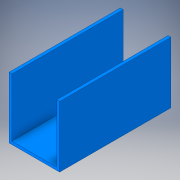
# Autodesk Inventor part: Hombro_base
Saved by Autodesk Inventor 2019 (Build 230136000, 136)
## iProperties
Created: 2020-02-08
Part Number: Hombro_base
Material: Generic
Document SubType Name: Modeling
Designer: Omar
Density: 1 g/cm^3
Appearance: Default
Author: Omar
Autodesk Inventor part; units mm, degrees
ref_plane "YZ Plane" through (0, 0, 0) normal (1, 0, 0) x (0, 1, 0)
ref_plane "XZ Plane" through (0, 0, 0) normal (0, 1, 0) x (-1, 0, 0)
ref_plane "XY Plane" through (0, 0, 0) normal (0, 0, 1) x (1, 0, 0)
sketch "Sketch1" plane through (0, 0, 0) normal (0, 1, 0) x (-1, 0, 0)
  line L0 (-25, 62.04) -> (25, 62.04)
  line L1 (25, 62.04) -> (25, -62.04)
  line L2 (25, -62.04) -> (-25, -62.04)
  line L3 (-25, -62.04) -> (-25, 62.04)
  line L4 (-25, 62.04) -> (25, -62.04) construction
  line L5 (25, 62.04) -> (-25, -62.04) construction
  circle A0 centre (0, 17.59) radius 5
  point P0 (0, 0)
  dimension "d0" = 50
  dimension "d1" = 124.08
  dimension "d2" = 10
  dimension "d3" = 44.45
  dimension "d4" = 25
  constraints: 12 end point, 2 midpoint, 2 parallel, 1 centre point, 1 horizontal, 1 perpendicular
  measures "d0" distance of L1.end L2.end
  measures "d1" distance of L0.end L1.end
  measures "d2" diameter of A0
  measures "d3" distance from line of L0 A0.centre
  measures "d4" distance from line of L1 A0.centre
extrude "Extrusion1" add sketch "Sketch1" along normal blind 3.18
sketch "Sketch4" plane through (0, 0, 0) normal (0, 1, 0) x (-1, 0, 0)
  circle A0 centre (0, 17.59) radius 5 projected
  line L0 (25, 62.04) -> (-25, 62.04) projected
  line L1 (-25, 62.04) -> (-25, -62.04) projected
  line L2 (-25, -62.04) -> (25, -62.04) projected
  line L3 (25, -62.04) -> (25, 62.04) projected
  line L4 (25, 62.04) -> (28.18, 62.04)
  line L5 (28.18, 62.04) -> (28.18, -62.04)
  line L6 (28.18, -62.04) -> (25, -62.04)
  line L7 (25, -62.04) -> (25, 62.04)
  line L8 (-25, 62.04) -> (-28.18, 62.04)
  line L9 (-28.18, 62.04) -> (-28.18, -62.04)
  line L10 (-28.18, -62.04) -> (-25, -62.04)
  line L11 (-25, -62.04) -> (-25, 62.04)
  point P0 (0, 0)
  dimension "d11" = 3.18
  dimension "d12" = 3.18
  constraints: 16 end point, 4 parallel, 2 horizontal, 2 perpendicular, 1 point on line
  measures "d11" distance of L5.end L6.end
  measures "d12" distance of L10.end L9.end
extrude "Extrusion3" add sketch "Sketch4" along normal blind 68.18 contours L4 L5 L6 L3 | L1 L10 L9 L8
body "Solid1"
